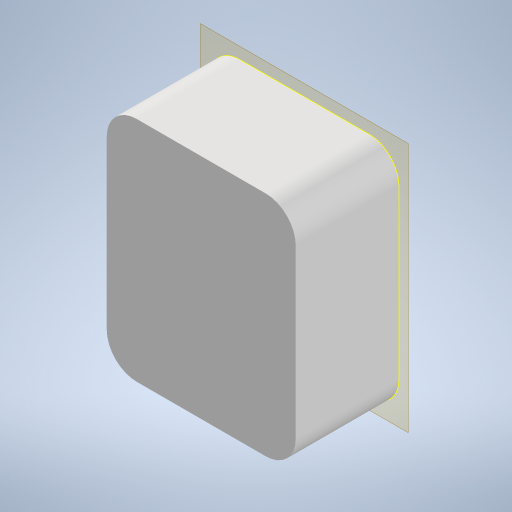
# Autodesk Inventor part: pumpswitch_top
Saved by Autodesk Inventor 2024.3 (Build 283343000, 343)
## iProperties
Created: 2024-10-21
Part Number: pumpswitch_top
Material: Generic
Document SubType Name: Modeling
Designer: atrus
Density: 1 g/cm^3
Appearance: Default
Author: atrus
Autodesk Inventor part; units mm, degrees
ref_plane "YZ Plane" through (0, 0, 0) normal (1, 0, 0) x (0, 1, 0)
ref_plane "XZ Plane" through (0, 0, 0) normal (0, 1, 0) x (-1, 0, 0)
ref_plane "XY Plane" through (0, 0, 0) normal (0, 0, 1) x (1, 0, 0)
ref_plane "Work Plane1" through (0, 0, 0) normal (0, 0, 1) x (1, 0, 0)
sketch "Sketch1" plane through (0, 0, 0) normal (0, 0, 1) x (1, 0, 0)
  arc A0 (22, 19.5) -> (15, 26.5) centre (15, 19.5) ccw projected
  line L0 (22, 19.5) -> (22, -19.5) projected
  arc A1 (15, -26.5) -> (22, -19.5) centre (15, -19.5) ccw projected
  line L1 (15, -26.5) -> (-15, -26.5) projected
  arc A2 (-22, -19.5) -> (-15, -26.5) centre (-15, -19.5) ccw projected
  line L2 (-22, -19.5) -> (-22, 19.5) projected
  arc A3 (-15, 26.5) -> (-22, 19.5) centre (-15, 19.5) ccw projected
  line L3 (-15, 26.5) -> (15, 26.5) projected
  line L4 (-20, -19.5) -> (-20, 19.5) projected
  arc A4 (-20, -19.5) -> (-15, -24.5) centre (-15, -19.5) ccw projected
  line L5 (-15, -24.5) -> (15, -24.5) projected
  arc A5 (15, -24.5) -> (20, -19.5) centre (15, -19.5) ccw projected
  line L6 (20, -19.5) -> (20, 19.5) projected
  arc A6 (20, 19.5) -> (15, 24.5) centre (15, 19.5) ccw projected
  line L7 (-15, 24.5) -> (15, 24.5) projected
  arc A7 (-15, 24.5) -> (-20, 19.5) centre (-15, 19.5) ccw projected
  circle A8 centre (-9, -4.5) radius 3.15 projected
extrude "Extrusion1" add sketch "Sketch1" along normal blind 22 contours L0 A1 L1 A2 L2 A3 L3 A0
sketch "Sketch2" plane through (0, 0, 0) normal (0, 0, -1) x (-1, 0, 0)
  line L0 (-22, -19.5) -> (-22, 19.5) projected
  arc A0 (-22, -19.5) -> (-15, -26.5) centre (-15, -19.5) ccw projected
  line L1 (15, -26.5) -> (-15, -26.5) projected
  arc A1 (15, -26.5) -> (22, -19.5) centre (15, -19.5) ccw projected
  line L2 (22, 19.5) -> (22, -19.5) projected
  arc A2 (22, 19.5) -> (15, 26.5) centre (15, 19.5) ccw projected
  line L3 (-15, 26.5) -> (15, 26.5) projected
  arc A3 (-15, 26.5) -> (-22, 19.5) centre (-15, 19.5) ccw projected
  arc A4 (15, -24.5) -> (20, -19.5) centre (15, -19.5) ccw projected
  line L4 (-15, -24.5) -> (15, -24.5) projected
  arc A5 (-20, -19.5) -> (-15, -24.5) centre (-15, -19.5) ccw projected
  line L5 (-20, 19.5) -> (-20, -19.5) projected
  arc A6 (-15, 24.5) -> (-20, 19.5) centre (-15, 19.5) ccw projected
  line L6 (15, 24.5) -> (-15, 24.5) projected
  arc A7 (20, 19.5) -> (15, 24.5) centre (15, 19.5) ccw projected
  line L7 (20, -19.5) -> (20, 19.5) projected
lip "Lip2" kind lip height 1 width 1 edges at (-18.5355, 23.0355, 0) (0, 24.5, 0) (18.5355, 23.0355, 0) (20, 0, 0) (18.5355, -23.0355, 0) (0, -24.5, 0) (-18.5355, -23.0355, 0) (-20, 0, 0) guide face at (21.3333, 6.5, 0)
sketch "Sketch6" plane through (0, 0, 22) normal (0, 0, 1) x (1, 0, 0)
  line L0 (15, 26.5) -> (-15, 26.5) projected
  arc A0 (22, 19.5) -> (15, 26.5) centre (15, 19.5) ccw projected
  line L1 (22, -19.5) -> (22, 19.5) projected
  arc A1 (15, -26.5) -> (22, -19.5) centre (15, -19.5) ccw projected
  line L2 (-15, -26.5) -> (15, -26.5) projected
  arc A2 (-22, -19.5) -> (-15, -26.5) centre (-15, -19.5) ccw projected
  line L3 (-22, 19.5) -> (-22, -19.5) projected
  arc A3 (-15, 26.5) -> (-22, 19.5) centre (-15, 19.5) ccw projected
  point P0 (0, 0)
extrude "Extrusion4" add sketch "Sketch6" along normal blind 2
sketch "Sketch7" plane through (0, 0, 22) normal (0, 0, -1) x (-1, 0, 0)
  circle A0 centre (9, -4.5) radius 1.7 projected
  circle A1 centre (9, -4.5) radius 3.5
  circle A2 centre (9, -4.5) radius 2.1
  point P0 (0, 0)
  dimension "d24" = 7
  dimension "d41" = 4.2
  constraints: 2 centre point, 2 coincident
  measures "d24" diameter of A1
  measures "d41" diameter of A2
ref_plane "Work Plane2" through (-17, -21.5, -0.0086) normal (0, 0, 1) x (1, 0, 0)
extrude "Extrusion5" add sketch "Sketch7" along normal up to surface (22.0086 mm away) contours A1
sketch "Sketch8" plane through (-15, -26.5, 0) normal (0, -1, 0) x (1, 0, 0)
  line L0 (23.3, 11.3813) -> (26.7, 11.3813) projected
  line L1 (27.7, 9.6813) -> (27.7, 3.2813) projected
  line L2 (2.241, 7.7913) -> (2.241, 5.0813) projected
  line L3 (28.2, 14.3813) -> (2.9035, 14.3813)
  line L4 (2.9035, 14.3813) -> (2.9035, -3)
  line L5 (2.9035, -3) -> (28.2, -3)
  line L6 (28.2, -3) -> (28.2, 14.3813)
  line L7 (0, -0.0086) -> (30, -0.0086) projected
  line L8 (22.3, 0.6813) -> (22.3, 9.6813) projected
  line L9 (18.7, 9.6813) -> (18.7, 3.2813) projected
  line L10 (13.3, 0.6813) -> (13.3, 9.6813) projected
  line L11 (7.7285, 7.7913) -> (7.7285, 0.5513) projected
  line L12 (3.9035, 0.5513) -> (3.9035, 7.7913) projected
  line L13 (0, -1) -> (30, -1) projected
  line L14 (8.7285, 14.3813) -> (12.3, 14.3813)
  line L15 (12.3, 14.3813) -> (12.3, -1)
  line L16 (12.3, -1) -> (8.7285, -1)
  line L17 (8.7285, -1) -> (8.7285, 14.3813)
  line L18 (14.2958, 14.3813) -> (17.7373, 14.3813)
  line L19 (17.7373, -0.0086) -> (14.2958, -0.0086)
  line L20 (19.7, 14.3813) -> (21.3, 14.3813)
  line L21 (21.3, 14.3813) -> (21.3, -0.0086)
  line L22 (21.3, -0.0086) -> (19.7, -0.0086)
  line L23 (19.7, -0.0086) -> (19.7, 14.3813)
  point P0 (15, 0)
  point P1 (28.2, 5.6906)
  point P2 (25, 11.3813)
  point P3 (2.9035, 5.6906)
  point P4 (2.241, 6.4363)
  point P5 (2.9035, -0.0086)
  point P6 (28.2, -0.0086)
  point P7 (7.7285, 4.1713)
  point P8 (13.3, 5.1813)
  point P9 (21.3, 7.1864)
  point P10 (12.3, -0.0086)
  point P11 (8.7285, -0.0086)
  dimension "d27" = 0.5
  dimension "d28" = 3
  dimension "d30" = 3
  dimension "d47" = 1
  dimension "d48" = 1
  dimension "d49" = 1
  dimension "d50" = 1
  dimension "d51" = 1
  constraints: 28 end point, 7 midpoint, 7 parallel, 6 point on line, 4 horizontal, 3 perpendicular
  measures "d27" distance from line of point (28.2, 5.691) L1
  measures "d28" distance from line of point (25, 11.381) L3
  measures "d30" distance from line of L5 point (15, 0)
  measures "d47" distance between parallel lines of L4 L12
  measures "d48" distance from line of L17 point (7.729, 4.171)
  measures "d49" distance from line of point (13.3, 5.181) L15
  measures "d50" distance between parallel lines of L9 L23
  measures "d51" distance from line of L8 point (21.3, 7.186)
extrude "Extrusion6" cut sketch "Sketch8" against normal blind 10 contours L6 L7 L21 L3 | L23 L7 L15 L3 | L7 L4 L3 L17
sketch "Sketch9" plane through (-9, -4.5, -0.0086) normal (0, 0, -1) x (-1, 0, 0)
  line L0 (6, -5) -> (11, -5) projected
  line L1 (6, -5) -> (6, -15) projected
  line L2 (6, -15) -> (11, -15) projected
  line L3 (11, -15) -> (11, -5) projected
  line L4 (-24, -5) -> (-29, -5) projected
  line L5 (-24, -15) -> (-24, -5) projected
  line L6 (-29, -15) -> (-24, -15) projected
  line L7 (11, 14) -> (6, 14) projected
  line L8 (6, 24) -> (6, 14) projected
  line L9 (11, 24) -> (6, 24) projected
  line L10 (11, 14) -> (11, 24) projected
  line L11 (-24, 24) -> (-29, 24) projected
  line L12 (-24, 14) -> (-24, 24) projected
  line L13 (-29, 14) -> (-24, 14) projected
  line L14 (-29, 24) -> (-29, 14) projected
  line L15 (-29, -5) -> (-29, -15) projected
  point P0 (-9, 4.5)
extrude "Extrusion7" add sketch "Sketch9" against normal up to surface (24.0086 mm away)
sketch "Sketch10" plane through (-9, -4.5, -0.0086) normal (0, 0, -1) x (-1, 0, 0)
  line L0 (11, 24) -> (6, 24) projected
  line L1 (6, 14) -> (11, 14) projected
  line L2 (11, 24) -> (8.2, 24)
  line L3 (8.2, 24) -> (8.2, 14)
  line L4 (8.2, 14) -> (11, 14)
  line L5 (11, 14) -> (11, 24)
  line L6 (-29, -15) -> (-29, 24) projected
  line L7 (-29, -5) -> (-26.2, -5)
  line L8 (-26.2, -5) -> (-26.2, -15)
  line L9 (-26.2, -15) -> (-29, -15)
  line L10 (-29, -15) -> (-29, -5)
  line L11 (11, -5) -> (6, -5) projected
  line L12 (6, -15) -> (11, -15) projected
  line L13 (11, -5) -> (8.2, -5)
  line L14 (8.2, -5) -> (8.2, -15)
  line L15 (8.2, -15) -> (11, -15)
  line L16 (11, -15) -> (11, -5)
  line L17 (-29, 14) -> (-24, 14) projected
  line L18 (-24, 24) -> (-29, 24) projected
  line L19 (-29, 14) -> (-26.2, 14)
  line L20 (-26.2, 14) -> (-26.2, 24)
  line L21 (-26.2, 24) -> (-29, 24)
  line L22 (-29, 24) -> (-29, 14)
  line L23 (-24, -5) -> (-29, -5) projected
  point P0 (-9, 4.5)
  point P1 (-27.6, -5)
  dimension "d42" = 2.8
  dimension "d44" = 2.8
  constraints: 32 end point, 8 parallel, 5 point on line, 4 horizontal, 4 perpendicular, 2 collinear, 1 midpoint
  measures "d42" distance between parallel lines of L5 L3
  measures "d44" distance between parallel lines of L10 L8
extrude "Extrusion8" add sketch "Sketch10" along normal blind 1.5
body "Solid1"
